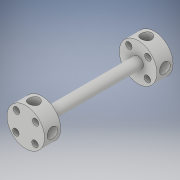
# Autodesk Inventor part: SweeperHub
Saved by Autodesk Inventor 2019 (Build 230136000, 136)
## iProperties
Created: 2018-12-01
Part Number: SweeperHub
Material: Generic
Document SubType Name: Modeling
Designer: User
Density: 1 g/cm^3
Appearance: Default
Author: User
Autodesk Inventor part; units mm, degrees
ref_plane "YZ Plane" through (0, 0, 0) normal (1, 0, 0) x (0, 1, 0)
ref_plane "XY Plane" through (0, 0, 0) normal (0, 0, 1) x (1, 0, 0)
sketch "Sketch2" plane through (0, 0, 0) normal (0, 0, 1) x (1, 0, 0)
  line L0 (0, 0) -> (3.175, -3.175) projected
  circle A0 centre (0, 0) radius 11.1125
  dimension "d6" = 22.225
  constraints: 1 centre point, 1 coincident
  measures "d6" diameter of A0
extrude "Extrusion2" add sketch "Sketch2" along normal mid plane 9.525
sketch "Sketch6" plane through (0, 0, 4.7625) normal (0, 0, 1) x (1, 0, 0)
  circle A0 centre (0, 0) radius 3.175
  dimension "d17" = 6.35
  constraints: 1 centre point, 1 coincident
  measures "d17" diameter of A0
extrude "Extrusion3" add sketch "Sketch6" along normal blind 28.448
sketch "Sketch7" plane through (0, 0, 4.7625) normal (0, 0, 1) x (1, 0, 0)
  circle A0 centre (0, 0) radius 3.175 projected
  line L0 (5.8251, 5.4849) -> (0.0652, -0.2751)
  line L1 (0, 0) -> (5.491, 0)
  dimension "d20" = 8.001
  dimension "d42" = 45
  constraints: 4 end point, 1 horizontal
  measures "d20" distance of point (0, 0) L0.start
  measures "d42" angle of L1 L0
hole "Hole2" at (5.8251, 5.4849, 4.7625) direction (0, 0, -1) diameter 3.81 end through all
pattern_circular "Circular Pattern2" count 4 over 360 about axis through (0, 0, 4.7625) along (0, 0, 1) of "Hole2"
ref_plane "Work Plane2" through (0, 11.1125, 0) normal (0, 1, 0) x (-1, 0, 0)
sketch "Sketch8" plane through (0, 11.1125, 0) normal (0, 1, 0) x (-1, 0, 0)
  point P0 (0, 0)
  point P1 (0, 0)
  constraints: 1 coincident
hole "Hole3" at (0, 11.1125, 0) direction (0, -1, 0) diameter 6.35 end through all
pattern_circular "Circular Pattern3" count 4 over 360 about axis through (0, 0, 4.7625) along (0, 0, 1) of "Hole3"
mirror "Mirror1" about plane through (0, 0, 33.2105) normal (0, 0, 1) of "Extrusion2", "Hole2", "Circular Pattern2", "Extrusion3", "Hole3", "Circular Pattern3"
body "Solid1"
